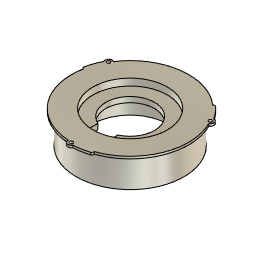
外壳3 v18 (Autodesk Fusion 360 design; units mm, degrees)
Autodesk Fusion 360 part; units mm, degrees
note: some values were not read from the file. Set by a fixed rule: which sketch regions a step uses.
sketch "草图1" plane through (0, 0, 0) normal (0, 0, 1) x (1, 0, 0)
  line L0 (28.4627, -32.3648) -> (28.4702, -32.3737)
  line L1 (41.5939, -11.2943) -> (41.768, -11.325)
  arc A0 (14.7507, -46.3074) -> (13.8402, -43.4489) centre (14.2954, -44.8782) ccw construction
  line L2 (-28.4627, -32.3648) -> (-28.4702, -32.3737)
  circle A1 centre (0, -47.1) radius 1.4
  line L3 (43.1, 0) -> (48, 0) construction
  line L4 (0, -43.1) -> (0, -51.1) construction
  arc A2 (2.5554, -45.5283) -> (2.6381, -48.5283) centre (0, -47.1) ccw construction
  circle A3 centre (0, 0) radius 44.72 construction
  arc A4 (2.6381, -48.5283) -> (14.7507, -46.3074) centre (0, 0) ccw construction
  line L5 (-30.5781, -30.3742) -> (-30.6917, -30.5096)
  line L6 (-41.5939, -11.2943) -> (-41.768, -11.325)
  line L7 (30.5781, -30.3742) -> (30.6917, -30.5096)
  line L8 (42.2601, -8.467) -> (42.2716, -8.469)
  line L9 (-42.2601, -8.467) -> (-42.2716, -8.469)
  line L10 (0.9, -43.0906) -> (0.9, -43.1)
  arc A5 (2.5554, -45.5283) -> (13.8402, -43.4489) centre (0, 0) ccw construction
  line L11 (-0.9, -43.0906) -> (-0.9, -43.1)
  circle A6 centre (0, 0) radius 43.1
  arc A7 (40.7077, 26.5489) -> (32.728, 35.9282) centre (0, 0) ccw construction
  line L12 (11.0158, 41.6685) -> (11.0763, 41.8346)
  line L13 (13.7974, 40.8319) -> (13.8014, 40.8428)
  line L14 (36.8676, 22.3247) -> (36.8757, 22.3294)
  arc A8 (32.728, 35.9282) -> (30.7078, 33.7104) centre (31.7179, 34.8193) ccw construction
  circle A9 centre (40.7898, 23.55) radius 1.4
  circle A10 centre (-40.7898, 23.55) radius 1.4
  line L15 (-15.6751, 9.05) -> (-16.3679, 9.45) construction
  arc A11 (38.151, 24.9772) -> (30.7078, 33.7104) centre (0, 0) ccw construction
  line L16 (-13.7974, 40.8319) -> (-13.8014, 40.8428)
  line L17 (37.7676, 20.7659) -> (37.7757, 20.7706)
  arc A12 (-40.7064, 20.5512) -> (-44.548, 9.7385) centre (0, 0) ccw construction
  arc A13 (-47.4788, 10.3792) -> (-44.548, 9.7385) centre (-46.0134, 10.0589) ccw construction
  circle A14 centre (0, 0) radius 47.1 construction
  arc A15 (-43.3459, 21.9795) -> (-47.4788, 10.3792) centre (0, 0) ccw construction
  line L18 (-37.7676, 20.7659) -> (-37.7757, 20.7706)
  line L19 (-36.8676, 22.3247) -> (-36.8757, 22.3294)
  arc A16 (38.151, 24.9772) -> (40.7077, 26.5489) centre (40.7898, 23.55) ccw construction
  circle A17 centre (0, 0) radius 47.1 construction
  line L20 (-11.0158, 41.6685) -> (-11.0763, 41.8346)
  line L21 (-37.3257, 21.55) -> (-41.5692, 24) construction
  arc A18 (-40.7064, 20.5512) -> (-43.3459, 21.9795) centre (-40.7898, 23.55) ccw construction
  circle A19 centre (0, 0) radius 46.9
  arc A20 (32.5934, 35.7803) -> (30.8425, 33.8583) centre (31.7179, 34.8193) ccw
  arc A21 (38.3851, 24.9844) -> (30.8425, 33.8583) centre (0, 0) ccw
  arc A22 (38.3851, 24.9844) -> (40.6026, 26.3437) centre (40.7898, 23.55) ccw
  arc A23 (40.6026, 26.3437) -> (32.5934, 35.7803) centre (0, 0) ccw
  arc A24 (2.4446, -45.7347) -> (13.9009, -43.6395) centre (0, 0) ccw
  arc A25 (14.69, -46.1168) -> (13.9009, -43.6395) centre (14.2954, -44.8782) ccw
  arc A26 (2.5131, -48.3347) -> (14.69, -46.1168) centre (0, 0) ccw
  arc A27 (2.4446, -45.7347) -> (2.5131, -48.3347) centre (0, -47.1) ccw
  arc A28 (-47.2834, 10.3365) -> (-44.7434, 9.7812) centre (-46.0134, 10.0589) ccw
  arc A29 (-40.8297, 20.7503) -> (-44.7434, 9.7812) centre (0, 0) ccw
  arc A30 (-40.8297, 20.7503) -> (-43.1156, 21.991) centre (-40.7898, 23.55) ccw
  arc A31 (-43.1156, 21.991) -> (-47.2834, 10.3365) centre (0, 0) ccw
  circle A32 centre (0, 0) radius 19.5
  dimension "d43" = 1.8
  dimension "d44" = 6
  dimension "d45" = 3
  dimension "d46" = 2.8
  dimension "d47" = 2.8
  dimension "d48" = 2.8
  dimension "d49" = 86.2
  dimension "d53" = -0.2
  dimension "d54" = -0.2
  dimension "d55" = -0.2
  dimension "d56" = -0.2
  dimension "d57" = 39
  constraint coincident A1.centre A14
  constraint coincident A0.centre A14
  constraint tangent A0 A5
  constraint tangent A0 A4
  constraint concentric A1 A2
  constraint concentric A10 A18
  constraint concentric A9 A16
  constraint coincident L13.start A6
  constraint coincident L20.start A6
  constraint coincident L16.start A6
  constraint coincident L12.start A6
  constraint coincident L18.start A6
  constraint coincident L19.start A6
  constraint coincident L21.start A6
  constraint collinear L15 L21
  constraint coincident L9.start A6
  constraint coincident L6.start A6
  constraint coincident L5.start A6
  constraint coincident L2.start A6
  constraint coincident L14.start A6
  constraint coincident L17.start A6
  constraint coincident L11.start A6
  constraint coincident L4.start A6
  constraint coincident L10.start A6
  constraint coincident L1.start A6
  constraint coincident L8.start A6
  constraint coincident L7.start A6
  constraint coincident L0.start A6
  constraint concentric A6 A17
  constraint coincident A9.centre A17
  constraint concentric A5 A32
  measures "d43" distance of L10 L11
  measures "d44" diameter of A2
  measures "d45" diameter of A0
  measures "d46" diameter of A1
  measures "d47" diameter of A10
  measures "d48" diameter of A9
  measures "d49" diameter of A6
  measures "d57" diameter of A32
extrude "拉伸5" add sketch "草图1" along normal blind 1.8 contours A1 A19 A25 A26 A27 | A1 A19 A24 A25 A27 | A19 A20 A21 A22 A24 A25 A27 A28 A29 A30 | A10 A19 A28 A30 A31 | A10 A19 A28 A29 A30 | A9 A19 A20 A21 A22 | A9 A19 A20 A22 A23
extrude "拉伸6" add sketch "草图1" along normal up to surface (1.8 mm away) contours A6
sketch "草图3" plane through (0, 0, 1.8) normal (0, 0, 1) x (-1, 0, 0)
  circle A0 centre (0, 0) radius 19.5
  circle A1 centre (40.7898, -23.55) radius 1.4
  circle A2 centre (-40.7898, -23.55) radius 1.4
  circle A3 centre (0, 47.1) radius 1.4
  arc A4 (43.1156, -21.991) -> (47.2834, -10.3365) centre (0, 0) ccw
  arc A5 (47.2834, -10.3365) -> (46.0746, -8.7603) centre (46.0134, -10.0589) ccw
  arc A6 (46.0746, -8.7603) -> (2.7857, 46.8172) centre (0, 0) ccw
  arc A7 (2.7857, 46.8172) -> (-2.5131, 48.3347) centre (0, 47.1) ccw
  arc A8 (-2.5131, 48.3347) -> (-14.69, 46.1168) centre (0, 0) ccw
  arc A9 (-14.69, 46.1168) -> (-15.4506, 44.2819) centre (-14.2954, 44.8782) ccw
  arc A10 (-15.4506, 44.2819) -> (-41.9377, -20.9961) centre (0, 0) ccw
  arc A11 (-41.9377, -20.9961) -> (-40.6026, -26.3437) centre (-40.7898, -23.55) ccw
  arc A12 (-40.6026, -26.3437) -> (-32.5934, -35.7803) centre (0, 0) ccw
  arc A13 (-32.5934, -35.7803) -> (-30.6239, -35.5216) centre (-31.7179, -34.8193) ccw
  arc A14 (-30.6239, -35.5216) -> (39.152, -25.8211) centre (0, 0) ccw
  arc A15 (39.152, -25.8211) -> (43.1156, -21.991) centre (40.7898, -23.55) ccw
  circle A16 centre (0, 0) radius 29.75
  dimension "d64" = 59.5
  constraint coincident A0.centre A4.centre
  measures "d64" diameter of A16
sketch "草图4" plane through (0, 0, 0) normal (0, 0, -1) x (1, 0, 0)
  circle A0 centre (0, 0) radius 19.5
  circle A1 centre (-40.7898, -23.55) radius 1.4
  circle A2 centre (40.7898, -23.55) radius 1.4
  circle A3 centre (0, 47.1) radius 1.4
  arc A4 (-47.2834, -10.3365) -> (-43.1156, -21.991) centre (0, 0) ccw
  arc A5 (-43.1156, -21.991) -> (-39.152, -25.8211) centre (-40.7898, -23.55) ccw
  arc A6 (-39.152, -25.8211) -> (30.6239, -35.5216) centre (0, 0) ccw
  arc A7 (30.6239, -35.5216) -> (32.5934, -35.7803) centre (31.7179, -34.8193) ccw
  arc A8 (32.5934, -35.7803) -> (40.6026, -26.3437) centre (0, 0) ccw
  arc A9 (40.6026, -26.3437) -> (41.9377, -20.9961) centre (40.7898, -23.55) ccw
  arc A10 (41.9377, -20.9961) -> (15.4506, 44.2819) centre (0, 0) ccw
  arc A11 (15.4506, 44.2819) -> (14.69, 46.1168) centre (14.2954, 44.8782) ccw
  arc A12 (14.69, 46.1168) -> (2.5131, 48.3347) centre (0, 0) ccw
  arc A13 (2.5131, 48.3347) -> (-2.7857, 46.8172) centre (0, 47.1) ccw
  arc A14 (-2.7857, 46.8172) -> (-46.0746, -8.7603) centre (0, 0) ccw
  arc A15 (-46.0746, -8.7603) -> (-47.2834, -10.3365) centre (-46.0134, -10.0589) ccw
  circle A16 centre (0, 0) radius 43.1
  dimension "d65" = 86.2
  constraint coincident A0.centre A4.centre
  measures "d65" diameter of A16
extrude "拉伸8" add sketch "草图4" along normal blind 18 contours A16
extrude "拉伸9" cut sketch "草图3" against normal blind 5.5 contours A16
sketch "草图5" plane through (0, 0, -3.7) normal (0, 0, 1) x (-1, 0, 0)
  circle A0 centre (0, 0) radius 19.5
  circle A1 centre (0, 0) radius 29.75
  line L0 (0.0358, 19.5) -> (0.0358, 29.75)
  line L1 (8.0358, 17.7673) -> (8.0358, 28.6442)
  line L2 (-7.9642, 17.7673) -> (-7.9642, 28.6642)
  constraint coincident A0 L0.start
  constraint coincident A1 L0.end
  constraint vertical L0
  constraint coincident A0 L1.start
  constraint symmetric L0 L1.start L2.start
  constraint coincident A1 L2.end
  constraint coincident A1 L1.end
extrude "拉伸10" cut sketch "草图5" against normal blind 20 contours A0 A1 L0 L1 | A0 A1 L0 L2
sketch "草图6" plane through (0, 0, -18) normal (0, 0, -1) x (1, 0, 0)
  circle A0 centre (0, 0) radius 43.1
  line L0 (-8.0358, 17.7673) -> (-8.0358, 28.6442)
  arc A1 (7.9642, 28.6642) -> (-8.0358, 28.6442) centre (0, 0) ccw
  line L1 (7.9642, 28.6642) -> (7.9642, 17.7995)
  arc A2 (-8.0358, 17.7673) -> (7.9642, 17.7995) centre (0, 0) ccw
  circle A3 centre (0, 0) radius 35
  circle A4 centre (0, -35) radius 1.31
  circle A5 centre (35, 0) radius 1.31
  circle A6 centre (0, 35) radius 1.31
  circle A7 centre (-35, 0) radius 1.31
  dimension "d73" = 70
  dimension "d74" = 2.62
  dimension "d76" = 360
  constraint coincident A0.centre A1.centre
  constraint coincident A3 A4.centre
  measures "d73" diameter of A3
  measures "d74" diameter of A4
extrude "拉伸11" cut sketch "草图6" against normal blind 8 contours A3 A5 | A3 A5 | A3 A6 | A3 A6 | A3 A4 | A3 A4 | A3 A7 | A3 A7
sketch "草图7" plane through (0, 0, -18) normal (0, 0, -1) x (1, 0, 0)
  circle A0 centre (35, 0) radius 1.31
  circle A1 centre (-35, 0) radius 1.31
  circle A2 centre (0, -35) radius 1.31
  circle A3 centre (0, 35) radius 1.31
  circle A4 centre (0, 0) radius 43.1
  line L0 (-8.0358, 17.7673) -> (-8.0358, 28.6442)
  arc A5 (7.9642, 28.6642) -> (-8.0358, 28.6442) centre (0, 0) ccw
  line L1 (7.9642, 28.6642) -> (7.9642, 17.7995)
  arc A6 (-8.0358, 17.7673) -> (7.9642, 17.7995) centre (0, 0) ccw
  circle A7 centre (0, 0) radius 30
  dimension "d79" = 60
  constraint coincident A4.centre A5.centre
  measures "d79" diameter of A7
extrude "拉伸12" cut sketch "草图7" against normal blind 10 contours A7
extrude "拉伸13" add 1 faces at (34.9911, 7.617, -18) along direction (0, 0, -1) blind 6
